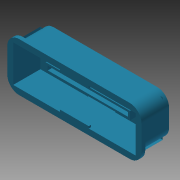
# Autodesk Inventor part: Socket(ellipse Insert)
Saved by Autodesk Inventor 2015 (Build 190159000, 159)
## iProperties
Created: 2014-10-29
Part Number: Socket(ellipse Insert)
Material: Generic
Document SubType Name: Modeling
Designer: cearhart275
Density: 1 g/cm^3
Appearance: Turquoise
Author: cearhart275
Autodesk Inventor part; units mm, degrees
ref_plane "YZ Plane" through (0, 0, 0) normal (1, 0, 0) x (0, 1, 0)
ref_plane "XZ Plane" through (0, 0, 0) normal (0, 1, 0) x (-1, 0, 0)
ref_plane "XY Plane" through (0, 0, 0) normal (0, 0, 1) x (1, 0, 0)
sketch "Sketch1" plane through (0, 0, 0) normal (0, 0, 1) x (1, 0, 0)
  line L0 (0, 0) -> (60.7568, 0)
  line L1 (60.7568, 0) -> (60.7568, 21.971)
  line L2 (60.7568, 21.971) -> (0, 21.971)
  line L3 (0, 21.971) -> (0, 0)
  dimension "d0" = 60.7568
  dimension "d1" = 21.971
  constraints: 8 end point, 2 parallel, 1 horizontal, 1 perpendicular
  measures "d0" distance of L1.end L2.end
  measures "d1" distance of L0.end L1.end
extrude "Extrusion1" add sketch "Sketch1" along normal blind 14.1199
sketch "Sketch2" plane through (0, 0, 14.1199) normal (0, 0, 1) x (1, 0, 0)
  line L0 (0, 21.971) -> (60.7568, 21.971) construction
  line L1 (60.7568, 21.971) -> (60.7568, 0) construction
  line L2 (60.7568, 0) -> (0, 0) construction
  line L3 (0, 0) -> (0, 21.971) construction
  line L4 (58.0923, 19.3065) -> (2.6645, 19.3065)
  line L5 (2.6645, 19.3065) -> (2.6645, 2.6645)
  line L6 (2.6645, 2.6645) -> (58.0923, 2.6645)
  line L7 (58.0923, 2.6645) -> (58.0923, 19.3065)
  point P0 (0, 0)
  dimension "d4" = 2.6645
  constraints: 16 end point, 4 parallel, 2 perpendicular, 1 horizontal, 3 other
  measures "d4" distance between parallel lines of L0 L4
extrude "Extrusion2" cut sketch "Sketch2" against normal blind 12.319
sketch "Sketch3" plane through (0, 0, 0) normal (0, 0, -1) x (-1, 0, 0)
  line L0 (-60.7568, 21.971) -> (0, 21.971)
  line L1 (0, 21.971) -> (0, 0)
  line L2 (0, 0) -> (-60.7568, 0)
  line L3 (-60.7568, 0) -> (-60.7568, 21.971)
  line L4 (-1.651, 20.32) -> (-59.1058, 20.32)
  line L5 (-59.1058, 20.32) -> (-59.1058, 1.651)
  line L6 (-59.1058, 1.651) -> (-1.651, 1.651)
  line L7 (-1.651, 1.651) -> (-1.651, 20.32)
  dimension "d7" = 1.651
  constraints: 16 end point, 4 parallel, 2 perpendicular, 1 horizontal, 3 other
  measures "d7" distance between parallel lines of L0 L4
extrude "Extrusion3" cut sketch "Sketch3" against normal blind 12.4206
fillet "Fillet1" radius 5.334 8 edges at (0, 21.971, 13.2702) (60.7568, 21.971, 13.2702) (60.7568, 0, 13.2702) (0, 0, 13.2702) (1.651, 20.32, 6.2103) (59.1058, 20.32, 6.2103) (59.1058, 1.651, 6.2103) (1.651, 1.651, 6.2103)
sketch "Sketch4" plane through (0, 0, 1.8009) normal (0, 0, 1) x (1, 0, 0)
  line L0 (11.3005, 12.8295) -> (49.4563, 12.8295)
  line L1 (49.4563, 12.8295) -> (49.4563, 9.1415)
  line L2 (49.4563, 9.1415) -> (11.3005, 9.1415)
  line L3 (11.3005, 9.1415) -> (11.3005, 12.8295)
  line L4 (2.6645, 2.6645) -> (2.6645, 19.3065) projected
  line L5 (58.0923, 19.3065) -> (58.0923, 2.6645) projected
  line L6 (2.6645, 19.3065) -> (58.0923, 19.3065) projected
  line L7 (58.0923, 2.6645) -> (2.6645, 2.6645) projected
  line L8 (48.5419, 11.9151) -> (12.2149, 11.9151)
  line L9 (12.2149, 11.9151) -> (12.2149, 10.0559)
  line L10 (12.2149, 10.0559) -> (48.5419, 10.0559)
  line L11 (48.5419, 10.0559) -> (48.5419, 11.9151)
  point P0 (0, 0)
  dimension "d12" = 8.636
  dimension "d13" = 8.636
  dimension "d14" = 6.477
  dimension "d15" = 6.477
  dimension "d16" = 0.9144
  constraints: 16 end point, 4 parallel, 2 perpendicular, 1 horizontal, 3 other
  measures "d12" distance between parallel lines of L3 L4
  measures "d13" distance between parallel lines of L5 L1
  measures "d14" distance between parallel lines of L6 L0
  measures "d15" distance between parallel lines of L2 L7
  measures "d16" distance between parallel lines of L0 L8
extrude "Extrusion4" add sketch "Sketch4" along normal blind 6.223 contours L0 L1 L2 L3
sketch "Sketch5" plane through (0, 0, 1.8009) normal (0, 0, 1) x (1, 0, 0)
  line L0 (58.0923, 2.6645) -> (2.6645, 2.6645) projected
  line L1 (24.1275, 3.6297) -> (36.6293, 3.6297)
  line L2 (36.6293, 3.6297) -> (36.6293, 2.6645)
  line L3 (36.6293, 2.6645) -> (24.1275, 2.6645)
  line L4 (24.1275, 2.6645) -> (24.1275, 3.6297)
  line L5 (2.6645, 19.3065) -> (58.0923, 19.3065) projected
  line L6 (24.1275, 19.3065) -> (36.6293, 19.3065)
  line L7 (36.6293, 19.3065) -> (36.6293, 18.3413)
  line L8 (36.6293, 18.3413) -> (24.1275, 18.3413)
  line L9 (24.1275, 18.3413) -> (24.1275, 19.3065)
  line L10 (2.6645, 2.6645) -> (2.6645, 19.3065) projected
  line L11 (58.0923, 19.3065) -> (58.0923, 2.6645) projected
  point P0 (0, 0)
  dimension "d19" = 21.463
  dimension "d20" = 21.463
  dimension "d21" = 21.463
  dimension "d22" = 21.463
  dimension "d23" = 0.9652
  dimension "d24" = 0.9652
  constraints: 16 end point, 4 parallel, 2 horizontal, 2 perpendicular, 2 point on line
  measures "d19" distance between parallel lines of L10 L9
  measures "d20" distance between parallel lines of L11 L7
  measures "d21" distance between parallel lines of L10 L4
  measures "d22" distance between parallel lines of L11 L2
  measures "d23" distance of L3.end L1.start
  measures "d24" distance of L8.end L6.start
extrude "Extrusion5" cut sketch "Sketch5" against normal blind 6.223 contours L0 L4 L1 L2 | L7 L8 L9 L5
sketch "Sketch6" plane through (2.6645, 2.6645, 14.1199) normal (0, 1, 0) x (1, 0, 0)
  line L0 (55.4279, 0) -> (0, 0) construction
  line L1 (21.2344, 0) -> (34.1935, 0)
  line L2 (34.1935, 0) -> (34.1935, 0.9652)
  line L3 (34.1935, 0.9652) -> (21.2344, 0.9652)
  line L4 (21.2344, 0.9652) -> (21.2344, 0)
  line L5 (0, 0) -> (0, 12.319) construction
  line L6 (55.4279, 0) -> (55.4279, 12.319) construction
  point P0 (-2.6645, 14.1199)
  dimension "d27" = 21.2344
  dimension "d28" = 21.2344
  dimension "d29" = 0.9652
  constraints: 10 end point, 2 horizontal, 2 parallel, 1 perpendicular, 1 point on line
  measures "d27" distance between parallel lines of L5 L4
  measures "d28" distance between parallel lines of L6 L2
  measures "d29" distance of L3.end L1.start
extrude "Extrusion6" add sketch "Sketch6" along normal up to next
sketch "Sketch7" plane through (0, 0, 14.1199) normal (0, 0, 1) x (1, 0, 0)
  line L0 (23.8989, 2.6645) -> (23.8989, 19.3065) projected
  line L1 (36.8579, 2.6645) -> (36.8579, 19.3065) projected
  line L2 (23.8989, 3.5789) -> (36.8579, 3.5789)
  line L3 (36.8579, 3.5789) -> (36.8579, 18.3921)
  line L4 (36.8579, 18.3921) -> (23.8989, 18.3921)
  line L5 (23.8989, 18.3921) -> (23.8989, 3.5789)
  line L6 (36.8579, 19.3065) -> (58.0923, 19.3065) projected
  line L7 (58.0923, 2.6645) -> (36.8579, 2.6645) projected
  point P0 (0, 0)
  dimension "d32" = 0.9144
  dimension "d33" = 0.9144
  constraints: 8 end point, 2 parallel, 2 point on line, 1 horizontal, 1 perpendicular
  measures "d32" distance between parallel lines of L6 L4
  measures "d33" distance between parallel lines of L7 L2
extrude "Extrusion7" cut sketch "Sketch7" against normal up to next
equation "\"d13\" = d12"
equation "\"d15\" = d14"
equation "\"d20\" = d19"
equation "\"d21\" = d19"
equation "\"d22\" = d20"
equation "\"d24\" = d23"
equation "\"d28\" = d27"
equation "\"d33\" = d32"
body "Solid1"
